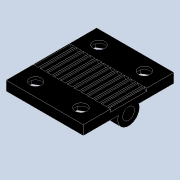
# Autodesk Inventor part: Y Axis Belt Adjustable Grip Plate
Saved by Autodesk Inventor 2022 (Build 260153000, 153)
## iProperties
Created: 2021-10-19
Part Number: Y Axis Belt Adjustable Grip Plate
Material: Generic
Document SubType Name: Modeling
Designer: Coy
Density: 1 g/cm^3
Appearance: Anodized - Black
Author: Coy
Autodesk Inventor part; units mm, degrees
ref_plane "YZ Plane" through (0, 0, 0) normal (1, 0, 0) x (0, 1, 0)
ref_plane "XZ Plane" through (0, 0, 0) normal (0, 1, 0) x (-1, 0, 0)
ref_plane "XY Plane" through (0, 0, 0) normal (0, 0, 1) x (1, 0, 0)
sketch "Sketch1" plane through (0, 0, 0) normal (0, 0, 1) x (1, 0, 0)
  line L0 (-34.1, 30.847) -> (0, 30.847)
  line L1 (0, 33.247) -> (-34.1, 33.247)
  arc A0 (-0.8878, 31.7995) -> (0, 30.847) centre (0, 31.737) ccw
  line L2 (-3, 33.247) -> (-3, 30.847) construction
  line L3 (-7.3, 30.847) -> (-2.1, 30.847)
  line L4 (0, 30.847) -> (-34.1, 30.847) construction
  line L5 (0, 33.247) -> (0, 30.847)
  arc A1 (-3, 30.847) -> (-2.1122, 31.7995) centre (-3, 31.737) ccw
  line L6 (-34.1, 32.067) -> (-3, 32.067) construction
  line L7 (-1.8628, 32.067) -> (-1.1372, 32.067)
  arc A2 (-1.8628, 32.067) -> (-2.1122, 31.7995) centre (-1.8628, 31.817) ccw
  arc A3 (-0.8878, 31.7995) -> (-1.1372, 32.067) centre (-1.1372, 31.817) ccw
  arc A4 (-3.8878, 31.7995) -> (-3, 30.847) centre (-3, 31.737) ccw
  arc A5 (-3.8878, 31.7995) -> (-4.1372, 32.067) centre (-4.1372, 31.817) ccw
  line L8 (-4.1372, 32.067) -> (-4.8628, 32.067)
  arc A6 (-4.8628, 32.067) -> (-5.1122, 31.7995) centre (-4.8628, 31.817) ccw
  arc A7 (-6, 30.847) -> (-5.1122, 31.7995) centre (-6, 31.737) ccw
  line L9 (-6, 33.247) -> (-6, 30.847) construction
  line L10 (-9, 33.247) -> (-9, 30.847) construction
  arc A8 (-9, 30.847) -> (-8.1122, 31.7995) centre (-9, 31.737) ccw
  arc A9 (-7.8628, 32.067) -> (-8.1122, 31.7995) centre (-7.8628, 31.817) ccw
  line L11 (-7.1372, 32.067) -> (-7.8628, 32.067)
  arc A10 (-6.8878, 31.7995) -> (-7.1372, 32.067) centre (-7.1372, 31.817) ccw
  arc A11 (-6.8878, 31.7995) -> (-6, 30.847) centre (-6, 31.737) ccw
  line L12 (-12, 33.247) -> (-12, 30.847) construction
  arc A12 (-12, 30.847) -> (-11.1122, 31.7995) centre (-12, 31.737) ccw
  arc A13 (-10.8628, 32.067) -> (-11.1122, 31.7995) centre (-10.8628, 31.817) ccw
  line L13 (-10.1372, 32.067) -> (-10.8628, 32.067)
  arc A14 (-9.8878, 31.7995) -> (-10.1372, 32.067) centre (-10.1372, 31.817) ccw
  arc A15 (-9.8878, 31.7995) -> (-9, 30.847) centre (-9, 31.737) ccw
  line L14 (-15, 33.247) -> (-15, 30.847) construction
  arc A16 (-15, 30.847) -> (-14.1122, 31.7995) centre (-15, 31.737) ccw
  arc A17 (-13.8628, 32.067) -> (-14.1122, 31.7995) centre (-13.8628, 31.817) ccw
  line L15 (-13.1372, 32.067) -> (-13.8628, 32.067)
  arc A18 (-12.8878, 31.7995) -> (-13.1372, 32.067) centre (-13.1372, 31.817) ccw
  arc A19 (-12.8878, 31.7995) -> (-12, 30.847) centre (-12, 31.737) ccw
  line L16 (-18, 33.247) -> (-18, 30.847) construction
  arc A20 (-18, 30.847) -> (-17.1122, 31.7995) centre (-18, 31.737) ccw
  arc A21 (-16.8628, 32.067) -> (-17.1122, 31.7995) centre (-16.8628, 31.817) ccw
  line L17 (-16.1372, 32.067) -> (-16.8628, 32.067)
  arc A22 (-15.8878, 31.7995) -> (-16.1372, 32.067) centre (-16.1372, 31.817) ccw
  arc A23 (-15.8878, 31.7995) -> (-15, 30.847) centre (-15, 31.737) ccw
  line L18 (-21, 33.247) -> (-21, 30.847) construction
  arc A24 (-21, 30.847) -> (-20.1122, 31.7995) centre (-21, 31.737) ccw
  arc A25 (-19.8628, 32.067) -> (-20.1122, 31.7995) centre (-19.8628, 31.817) ccw
  line L19 (-19.1372, 32.067) -> (-19.8628, 32.067)
  arc A26 (-18.8878, 31.7995) -> (-19.1372, 32.067) centre (-19.1372, 31.817) ccw
  arc A27 (-18.8878, 31.7995) -> (-18, 30.847) centre (-18, 31.737) ccw
  line L20 (-24, 33.247) -> (-24, 30.847) construction
  arc A28 (-24, 30.847) -> (-23.1122, 31.7995) centre (-24, 31.737) ccw
  arc A29 (-22.8628, 32.067) -> (-23.1122, 31.7995) centre (-22.8628, 31.817) ccw
  line L21 (-22.1372, 32.067) -> (-22.8628, 32.067)
  arc A30 (-21.8878, 31.7995) -> (-22.1372, 32.067) centre (-22.1372, 31.817) ccw
  arc A31 (-21.8878, 31.7995) -> (-21, 30.847) centre (-21, 31.737) ccw
  line L22 (-27, 33.247) -> (-27, 30.847) construction
  arc A32 (-27, 30.847) -> (-26.1122, 31.7995) centre (-27, 31.737) ccw
  arc A33 (-25.8628, 32.067) -> (-26.1122, 31.7995) centre (-25.8628, 31.817) ccw
  line L23 (-25.1372, 32.067) -> (-25.8628, 32.067)
  arc A34 (-24.8878, 31.7995) -> (-25.1372, 32.067) centre (-25.1372, 31.817) ccw
  arc A35 (-24.8878, 31.7995) -> (-24, 30.847) centre (-24, 31.737) ccw
  line L24 (-30, 33.247) -> (-30, 30.847) construction
  arc A36 (-30, 30.847) -> (-29.1122, 31.7995) centre (-30, 31.737) ccw
  arc A37 (-28.8628, 32.067) -> (-29.1122, 31.7995) centre (-28.8628, 31.817) ccw
  line L25 (-28.1372, 32.067) -> (-28.8628, 32.067)
  arc A38 (-27.8878, 31.7995) -> (-28.1372, 32.067) centre (-28.1372, 31.817) ccw
  arc A39 (-27.8878, 31.7995) -> (-27, 30.847) centre (-27, 31.737) ccw
  line L26 (-33, 33.247) -> (-33, 30.847) construction
  arc A40 (-33, 30.847) -> (-32.1122, 31.7995) centre (-33, 31.737) ccw
  arc A41 (-31.8628, 32.067) -> (-32.1122, 31.7995) centre (-31.8628, 31.817) ccw
  line L27 (-31.1372, 32.067) -> (-31.8628, 32.067)
  arc A42 (-30.8878, 31.7995) -> (-31.1372, 32.067) centre (-31.1372, 31.817) ccw
  arc A43 (-30.8878, 31.7995) -> (-30, 30.847) centre (-30, 31.737) ccw
  line L28 (-36, 33.247) -> (-36, 30.847) construction
  arc A44 (-36, 30.847) -> (-35.1122, 31.7995) centre (-36, 31.737) ccw
  arc A45 (-34.8628, 32.067) -> (-35.1122, 31.7995) centre (-34.8628, 31.817) ccw
  line L29 (-34.1372, 32.067) -> (-34.8628, 32.067)
  arc A46 (-33.8878, 31.7995) -> (-34.1372, 32.067) centre (-34.1372, 31.817) ccw
  arc A47 (-33.8878, 31.7995) -> (-33, 30.847) centre (-33, 31.737) ccw
  line L30 (-34.1, 30.847) -> (-34.1, 33.247)
  line L31 (-34.1, 30.847) -> (0, 30.847)
  line L32 (0, 30.847) -> (0, 27.847)
  line L33 (0, 27.847) -> (-34.1, 27.847)
  line L34 (-34.1, 27.847) -> (-34.1, 30.847)
  point P0 (0, 0)
  point P1 (0, 20)
  point P2 (-0.8266, 32.067)
  point P3 (-2.1734, 32.067)
  point P4 (-34.1, 32.0642)
  point P5 (-34.1, 32.0642)
  dimension "d4" = 2.4
  dimension "d5" = 1.78
  dimension "d6" = 3
  dimension "d7" = 1.78
  dimension "d8" = 0.25
  dimension "d9" = 0.25
  dimension "d10" = 3
  dimension "d12" = 3
  constraints: 98 point on circle, 70 end point, 48 centre point, 9 symmetric about line, 6 point on line, 6 tangent, 5 horizontal, 3 perpendicular, 2 parallel, 174 other
  measures "d4" distance between parallel lines of L0 L1
  measures "d5" diameter of A0
  measures "d6" distance between parallel lines of L5 L2
  measures "d7" diameter of A1
  measures "d8" radius of A2
  measures "d9" radius of A3
  measures "d10" distance of L9.start L10.start
  measures "d12" distance of L31.end L32.end
extrude "Extrusion1" add sketch "Sketch1" against normal blind 16 contours L30 A46 A47 L0 | L0 L32 L33 L34 | A40 A41 L27 A42 A43 L0 | A36 A37 L25 A38 A39 L0 | A32 A33 L23 A34 A35 L0 | L0 A1 A2 L7 A3 A0 | A28 A29 L21 A30 A31 L0 | A24 A25 L19 A26 A27 L0 | L0 A7 A6 L8 A5 A4 | A20 A21 L17 A22 A23 L0 | L0 A8 A9 L11 A10 A11 | A16 A17 L15 A18 A19 L0 | A12 A13 L13 A14 A15 L0
sketch "Sketch2" plane through (0, 27.847, 0) normal (1, 0, 0) x (0, 0, -1)
  line L0 (0, 0) -> (0, 3) projected
  line L1 (0, 0) -> (16, 0) projected
  line L2 (16, 3) -> (16, 0) projected
  line L3 (0, 3) -> (16, 3) projected
  line L4 (0, 0) -> (16, 0) construction
  line L5 (8, 0) -> (8, -9.1602) construction
  circle A0 centre (8, -1.5) radius 4.8
  circle A1 centre (8, -1.5) radius 2.6
  point P0 (0, -27.847)
  point P1 (5.8763, 0)
  point P2 (3.4404, 0)
  point P3 (12.5596, 0)
  point P4 (10.1237, 0)
  dimension "d15" = 9.6
  dimension "d16" = 1.5
  dimension "d17" = 5.2
  constraints: 2 centre point, 2 end point, 1 coincident, 1 midpoint, 1 point on line, 1 vertical
  measures "d15" diameter of A0
  measures "d16" distance from line of L1 A0.centre
  measures "d17" diameter of A1
extrude "Extrusion2" add sketch "Sketch2" against normal up to surface (34.1 mm away) contours L1 A1 A0
sketch "Sketch3" plane through (0, 27.847, 0) normal (1, 0, 0) x (0, 0, -1)
  arc A0 (5.8763, 0) -> (10.1237, 0) centre (8, -1.5) ccw projected
  line L0 (5.8763, 0) -> (10.1237, 0) projected
  circle A1 centre (8, -1.5) radius 2.6
  point P0 (0, -27.847)
  constraints: 1 coincident, 3 other
extrude "Extrusion3" cut sketch "Sketch3" against normal through all contours A1 L0
sketch "Sketch4" plane through (-34.1, 27.847, -16) normal (0, -1, 0) x (1, 0, 0)
  line L0 (33.21, 16) -> (34.1, 16) projected
  line L1 (34.1, 16) -> (0, 16)
  line L2 (0, 16) -> (0, 28)
  line L3 (0, 28) -> (34.1, 28)
  line L4 (34.1, 28) -> (34.1, 16)
  line L5 (34.1, 3.4404) -> (34.1, 0) projected
  line L6 (34.1, 0) -> (0, 0)
  line L7 (0, 0) -> (0, -12)
  line L8 (0, -12) -> (34.1, -12)
  line L9 (34.1, -12) -> (34.1, 0)
  line L10 (34.1, 22) -> (0, 22) construction
  line L11 (34.1, -6) -> (0, -6) construction
  line L12 (27.05, 22) -> (7.05, 22) construction
  line L13 (7.05, 22) -> (7.05, -6) construction
  line L14 (7.05, -6) -> (27.05, -6) construction
  line L15 (27.05, -6) -> (27.05, 22) construction
  line L16 (23, 24.3383) -> (27.05, 26.6765)
  line L17 (27.05, 26.6765) -> (31.1, 24.3383)
  line L18 (31.1, 24.3383) -> (31.1, 19.6617)
  line L19 (31.1, 19.6617) -> (27.05, 17.3235)
  line L20 (27.05, 17.3235) -> (23, 19.6617)
  line L21 (23, 19.6617) -> (23, 24.3383)
  line L22 (31.1, -3.6617) -> (31.1, -8.3383)
  line L23 (27.05, -1.3235) -> (31.1, -3.6617)
  line L24 (23, -3.6617) -> (27.05, -1.3235)
  line L25 (23, -8.3383) -> (23, -3.6617)
  line L26 (27.05, -10.6765) -> (23, -8.3383)
  line L27 (31.1, -8.3383) -> (27.05, -10.6765)
  line L28 (11.1, 24.3383) -> (11.1, 19.6617)
  line L29 (7.05, 26.6765) -> (11.1, 24.3383)
  line L30 (3, 24.3383) -> (7.05, 26.6765)
  line L31 (3, 19.6617) -> (3, 24.3383)
  line L32 (7.05, 17.3235) -> (3, 19.6617)
  line L33 (11.1, 19.6617) -> (7.05, 17.3235)
  line L34 (11.1, -3.6617) -> (11.1, -8.3383)
  line L35 (7.05, -1.3235) -> (11.1, -3.6617)
  line L36 (3, -3.6617) -> (7.05, -1.3235)
  line L37 (3, -8.3383) -> (3, -3.6617)
  line L38 (7.05, -10.6765) -> (3, -8.3383)
  line L39 (11.1, -8.3383) -> (7.05, -10.6765)
  point P0 (33.2122, 16)
  point P1 (23, 22)
  point P2 (23, -6)
  point P3 (3, 22)
  point P4 (3, -6)
  dimension "d22" = 12
  dimension "d23" = 12
  dimension "d24" = 4.05
  dimension "d25" = 20
  dimension "d26" = 7.05
  dimension "d29" = 28
  dimension "d32" = 20
  constraints: 76 end point, 6 parallel, 5 midpoint, 4 horizontal, 4 point on line, 3 perpendicular, 1 coincident, 1 vertical, 52 other
  measures "d22" distance of L1.end L2.end
  measures "d23" distance of L7.end L6.end
  measures "d24" distance from line of L12.start L21
  measures "d25" distance between parallel lines of L13 L15
  measures "d26" distance between parallel lines of L9 L15
  measures "d29" distance of L17.end L22.start
  measures "d32" distance of L17.end L28.start
extrude "Extrusion4" add sketch "Sketch4" against normal blind 3
sketch "Sketch5" plane through (-34.1, 30.847, -16) normal (0, 1, 0) x (1, 0, 0)
  line L0 (3, -19.6617) -> (3, -24.3383) construction
  line L1 (3, -22) -> (11.1, -22) construction
  line L2 (11.1, -24.3383) -> (11.1, -19.6617) construction
  line L3 (23, 3.6617) -> (23, 8.3383) construction
  line L4 (23, 6) -> (31.1, 6) construction
  line L5 (31.1, 8.3383) -> (31.1, 3.6617) construction
  line L6 (7.05, -22) -> (27.05, -22) construction
  line L7 (27.05, -22) -> (27.05, 6) construction
  line L8 (27.05, 6) -> (7.05, 6) construction
  line L9 (7.05, 6) -> (7.05, -22) construction
  circle A0 centre (7.05, -22) radius 2.6
  circle A1 centre (7.05, 6) radius 2.6
  circle A2 centre (27.05, -22) radius 2.6
  circle A3 centre (27.05, 6) radius 2.6
  line L10 (0, -16) -> (0, -28) projected
  line L11 (0, -16) -> (0, 0) projected
  line L12 (0, 12) -> (0, 0) projected
  line L13 (34.1, 12) -> (0, 12) projected
  line L14 (34.1, 0) -> (34.1, 12) projected
  line L15 (34.1, -16) -> (34.1, 0) projected
  line L16 (34.1, -28) -> (34.1, -16) projected
  line L17 (0, -28) -> (34.1, -28) projected
  line L18 (0, -28) -> (34.1, -28) projected
  line L19 (34.1, -28) -> (34.1, -16) projected
  line L20 (31.1, -16) -> (34.1, -16) projected
  line L21 (28.1, -16) -> (31.1, -16) projected
  line L22 (25.1, -16) -> (28.1, -16) projected
  line L23 (22.1, -16) -> (25.1, -16) projected
  line L24 (19.1, -16) -> (22.1, -16) projected
  line L25 (16.1, -16) -> (19.1, -16) projected
  line L26 (13.1, -16) -> (16.1, -16) projected
  line L27 (10.1, -16) -> (13.1, -16) projected
  line L28 (7.1, -16) -> (10.1, -16) projected
  line L29 (4.1, -16) -> (7.1, -16) projected
  line L30 (1.1, -16) -> (4.1, -16) projected
  line L31 (0, -16) -> (1.1, -16) projected
  line L32 (0, -16) -> (0, -28) projected
  line L33 (11.1, -19.6617) -> (11.1, -24.3383) projected
  line L34 (11.1, -24.3383) -> (7.05, -26.6765) projected
  line L35 (7.05, -26.6765) -> (3, -24.3383) projected
  line L36 (3, -24.3383) -> (3, -19.6617) projected
  line L37 (3, -19.6617) -> (7.05, -17.3235) projected
  line L38 (7.05, -17.3235) -> (11.1, -19.6617) projected
  line L39 (27.05, -26.6765) -> (23, -24.3383) projected
  line L40 (23, -24.3383) -> (23, -19.6617) projected
  line L41 (23, -19.6617) -> (27.05, -17.3235) projected
  line L42 (27.05, -17.3235) -> (31.1, -19.6617) projected
  line L43 (31.1, -19.6617) -> (31.1, -24.3383) projected
  line L44 (31.1, -24.3383) -> (27.05, -26.6765) projected
  line L45 (34.1, 12) -> (0, 12) projected
  line L46 (0, 12) -> (0, 0) projected
  line L47 (1.1, 0) -> (0, 0) projected
  line L48 (4.1, 0) -> (1.1, 0) projected
  line L49 (7.1, 0) -> (4.1, 0) projected
  line L50 (10.1, 0) -> (7.1, 0) projected
  line L51 (13.1, 0) -> (10.1, 0) projected
  line L52 (16.1, 0) -> (13.1, 0) projected
  line L53 (19.1, 0) -> (16.1, 0) projected
  line L54 (22.1, 0) -> (19.1, 0) projected
  line L55 (25.1, 0) -> (22.1, 0) projected
  line L56 (28.1, 0) -> (25.1, 0) projected
  line L57 (31.1, 0) -> (28.1, 0) projected
  line L58 (34.1, 0) -> (31.1, 0) projected
  line L59 (34.1, 0) -> (34.1, 12) projected
  line L60 (11.1, 8.3383) -> (11.1, 3.6617) projected
  line L61 (11.1, 3.6617) -> (7.05, 1.3235) projected
  line L62 (7.05, 1.3235) -> (3, 3.6617) projected
  line L63 (3, 3.6617) -> (3, 8.3383) projected
  line L64 (3, 8.3383) -> (7.05, 10.6765) projected
  line L65 (7.05, 10.6765) -> (11.1, 8.3383) projected
  line L66 (31.1, 8.3383) -> (31.1, 3.6617) projected
  line L67 (31.1, 3.6617) -> (27.05, 1.3235) projected
  line L68 (27.05, 1.3235) -> (23, 3.6617) projected
  line L69 (23, 3.6617) -> (23, 8.3383) projected
  line L70 (23, 8.3383) -> (27.05, 10.6765) projected
  line L71 (27.05, 10.6765) -> (31.1, 8.3383) projected
  dimension "d37" = 5.2
  dimension "d38" = 5.2
  dimension "d39" = 5.2
  dimension "d40" = 5.2
  constraints: 12 end point, 6 midpoint, 4 centre point, 4 coincident, 2 parallel, 1 horizontal, 1 perpendicular
  measures "d37" diameter of A0
  measures "d38" diameter of A1
  measures "d39" diameter of A2
  measures "d40" diameter of A3
extrude "Extrusion5" add sketch "Sketch5" along normal up to surface (1.22 mm away) contours L31 L30 L29 L28 L27 L26 L25 L24 L23 L22 L21 L20 L16 L17 L10 | L12 L13 L14 L58 L57 L56 L55 L54 L53 L52 L51 L50 L49 L48 L47 | L33 L34 L35 L36 L37 L38 | L39 L40 L41 L42 L43 L44 | L60 L61 L62 L63 L64 L65 | L66 L67 L68 L69 L70 L71
equation "\"d7\" = d5"
equation "\"d23\" = d22"
body "Solid1"
